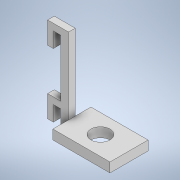
# Autodesk Inventor part: round_1_0_inchHoleV01
Saved by Autodesk Inventor 2020.2 (Build 242310000, 310)
## iProperties
Created: 2020-03-08
Part Number: round_1_0_inchHoleV01
Material: Generic
Document SubType Name: Modeling
Designer: robst
Density: 1 g/cm^3
Appearance: Default
Author: robst
Autodesk Inventor part; units mm, degrees
ref_plane "YZ Plane" through (0, 0, 0) normal (1, 0, 0) x (0, 1, 0)
ref_plane "XZ Plane" through (0, 0, 0) normal (0, 1, 0) x (-1, 0, 0)
ref_plane "XY Plane" through (0, 0, 0) normal (0, 0, 1) x (1, 0, 0)
sketch "Sketch1" plane through (0, 0, 0) normal (0, 0, 1) x (1, 0, 0)
  line L0 (0, 6.35) -> (0, 57.15)
  line L1 (0, 57.15) -> (-13.97, 57.15)
  line L2 (-13.97, 57.15) -> (-13.97, 55.245)
  line L3 (-10.16, 52.705) -> (-5.08, 52.705)
  line L4 (-5.08, 52.705) -> (-5.08, 14.605)
  line L5 (-5.08, 14.605) -> (-13.97, 14.605)
  line L6 (-13.97, 14.605) -> (-13.97, 12.7)
  line L7 (-10.16, 10.16) -> (-5.08, 10.16)
  line L8 (-5.08, 10.16) -> (-5.08, 0)
  line L9 (-5.08, 0) -> (0, 0)
  line L10 (-13.97, 55.245) -> (-13.97, 42.545)
  line L11 (-13.97, 42.545) -> (-10.16, 42.545)
  line L12 (-10.16, 42.545) -> (-10.16, 52.705)
  line L13 (-13.97, 12.7) -> (-13.97, 0)
  line L14 (-13.97, 0) -> (-10.16, 0)
  line L15 (-10.16, 0) -> (-10.16, 10.16)
  line L16 (0, 0) -> (38.1, 0)
  line L17 (38.1, 0) -> (38.1, 6.35)
  line L18 (38.1, 6.35) -> (0, 6.35)
  dimension "d0" = 10.16
  dimension "d1" = 38.1
  dimension "d2" = 4.445
  dimension "d3" = 4.445
  dimension "d4" = 5.08
  dimension "d6" = 5.08
  dimension "d7" = 3.81
  dimension "d8" = 10.16
  dimension "d9" = 10.16
  dimension "d10" = 38.1
  constraints: 38 end point, 11 perpendicular, 4 point on line, 3 vertical, 2 parallel
  measures "d0" distance of L7.end L8.end
  measures "d1" distance of L3.end L4.end
  measures "d2" distance between parallel lines of L5 L7
  measures "d3" distance between parallel lines of L1 L3
  measures "d4" distance between parallel lines of L4 L0
  measures "d6" distance between parallel lines of L12 L4
  measures "d7" distance between parallel lines of L10 L12
  measures "d8" distance from line of L11 L3.start
  measures "d9" distance from line of L14 L7.start
  measures "d10" distance of L9.end L16.end
extrude "Extrusion1" add sketch "Sketch1" along normal mid plane 4.445
sketch "Sketch2" plane through (0, 0, 0) normal (0, 0, 1) x (1, 0, 0)
  line L0 (0, 6.35) -> (38.1, 6.35) projected
  line L1 (0, 0) -> (38.1, 0)
  line L2 (38.1, 0) -> (38.1, 6.35)
  line L3 (38.1, 6.35) -> (0, 6.35)
  line L4 (0, 6.35) -> (0, 0)
  constraints: 8 end point, 2 parallel, 1 horizontal, 1 perpendicular
extrude "Extrusion2" add sketch "Sketch2" along normal mid plane 25.4
sketch "Sketch3" plane through (0, 6.35, 12.7) normal (0, 1, 0) x (1, 0, 0)
  circle A0 centre (19.05, 12.7) radius 6.35
  line L0 (0, 12.7) -> (38.1, 12.7) construction
  line L1 (38.1, 25.4) -> (38.1, 0) construction
  dimension "d15" = 12.7
  constraints: 2 end point, 1 centre point, 1 midpoint
  measures "d15" diameter of A0
extrude "Extrusion3" cut sketch "Sketch3" against normal through all
body "Solid1"
